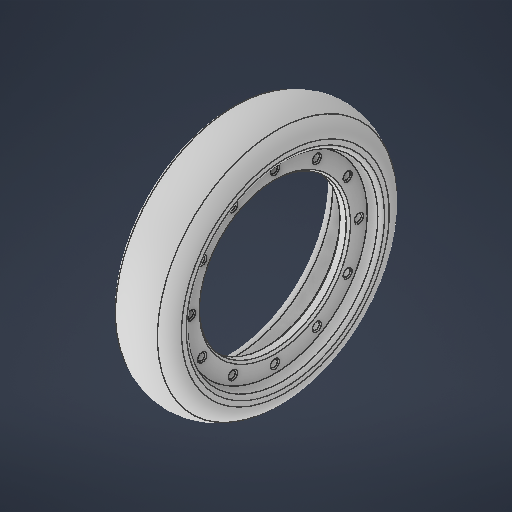
# Autodesk Inventor part: Колесо
Saved by Autodesk Inventor 2025 (Build 290162010, 162A)
## iProperties
Created: 2024-06-21
Part Number: Колесо
Material: Типовые
Document SubType Name: Modeling
Designer: Edward_Higgins
Density: 1 g/cm^3
Appearance: По умолчанию
Author: Edward_Higgins
Autodesk Inventor part; units mm, degrees
ref_plane "YZ Plane" through (0, 0, 0) normal (1, 0, 0) x (0, 1, 0)
ref_plane "XZ Plane" through (0, 0, 0) normal (0, 1, 0) x (-1, 0, 0)
ref_plane "XY Plane" through (0, 0, 0) normal (0, 0, 1) x (1, 0, 0)
sketch "Эскиз1" plane through (0, 0, 0) normal (0, 0, 1) x (1, 0, 0)
  line L0 (0, 0) -> (-61.3454, 0) construction
  line L1 (-14.2142, 60) -> (14.2142, 60) construction
  arc A0 (10, 56.9666) -> (-10, 56.9666) centre (0, 42) ccw
  arc A1 (14, 49.4833) -> (10, 56.9666) centre (5, 49.4833) ccw
  arc A2 (-10, 56.9666) -> (-13.9946, 49.7954) centre (-5, 49.4833) ccw
  line L2 (-3, 0) -> (-3, 9.8)
  line L3 (-3, 9.8) -> (-4.5, 9.8)
  line L4 (-4.5, 9.8) -> (-4.5, 12.1237)
  arc A3 (-3.7958, 13.6471) -> (-1, 18.6167) centre (-9.1319, 19.9203) ccw
  line L5 (4, 0) -> (4, 15)
  line L6 (-3, 4.05) -> (0, 4.05)
  line L7 (0, 4.05) -> (0, 0)
  arc A4 (-3.7958, 13.6471) -> (-4.5, 12.1237) centre (-2.5, 12.1237) ccw
  line L8 (4, 0) -> (-3, 0)
  line L9 (0, 4.05) -> (4, 4.05)
  arc A5 (-13.9946, 49.7954) -> (-9.8383, 46.3489) centre (-10.5856, 49.6771) ccw
  arc A6 (-1.893, 44.4558) -> (-9.8383, 46.3489) centre (-7.8016, 37.2774) ccw
  line L10 (14, 47.2203) -> (14, 49.4833)
  line L11 (9, 35) -> (4, 35)
  line L12 (4, 35) -> (4, 44)
  line L13 (-0.622, 44) -> (4, 44)
  line L14 (4, 15) -> (4, 43.7)
  arc A7 (-0.0249, 35.1197) -> (0, 35.6178) centre (-5, 35.6178) ccw
  arc A8 (-1.893, 44.4558) -> (-0.622, 44) centre (-0.622, 46) ccw
  line L15 (-9.8383, 46.3489) -> (-1.8928, 49.4771)
  arc A9 (0.1678, 45.7397) -> (-1.8928, 49.4771) centre (-1.1045, 47.4749) ccw
  line L16 (0.1678, 45.7397) -> (-0.622, 45.1605)
  line L17 (-0.622, 45.1605) -> (-0.622, 44)
  line L18 (9, 35) -> (9, 44)
  line L19 (9, 44) -> (12.684, 45.3409)
  arc A10 (12.684, 45.3409) -> (14, 47.2203) centre (12, 47.2203) ccw
  point P0 (0, 60)
  point P1 (-4.5, 13.1106)
  point P2 (-1.3791, 44)
  point P3 (0, 0)
  point P4 (14, 45.8199)
  dimension "d1" = 120
  dimension "d4" = 19.6
  dimension "d18" = 8.1
  dimension "d19" = 1.5
  dimension "d20" = 3
  dimension "d21" = 18
  dimension "d22" = 7
  dimension "d24" = 9
  dimension "d26" = 2
  dimension "d27" = 3
  dimension "d46" = 10
  dimension "d47" = 30
  dimension "d83" = 2
  dimension "d106" = 88
  dimension "d118" = 5
  dimension "d119" = 9
  dimension "d120" = 70
  dimension "d121" = 2
  constraints: 40 end point, 25 point on circle, 14 tangent, 11 centre point, 9 point on line, 6 perpendicular, 5 vertical, 4 horizontal, 2 horizontal alignment, 1 equal radius, 1 midpoint, 1 vertical alignment
  measures "d1" diameter of L1 L0
  measures "d4" diameter of L3 L0
  measures "d18" diameter of L6 L0
  measures "d19" distance between parallel lines of L2 L4
  measures "d20" distance between parallel lines of L2 L7
  measures "d21" radius of A0
  measures "d22" distance between parallel lines of L5 L2
  measures "d24" radius of A1
  measures "d26" radius of A4
  measures "d27" distance from line of L0.start L2
  measures "d46" distance of A1.centre A2.centre
  measures "d47" diameter of L5.end L0
  measures "d83" radius of A8
  measures "d106" diameter of L13 L0
  measures "d118" distance between parallel lines of L18 L14
  measures "d119" distance of L11.start L18.end
  measures "d120" angle of L18 L19
  measures "d121" radius of A10
revolve "Вращение1" add sketch "Эскиз1" angle 360 about axis through (0, 0, 0) along (-1, 0, 0) contours A1 L10 A10 L19 L18 L11 L12 L13 L17 L16 A9 L15 A5 A2 A0 | L15 A9 L16 L17 A8 A6
sketch "Эскиз8" plane through (14, 0, 0) normal (1, 0, 0) x (0, 0, -1)
  circle A0 centre (0, -40) radius 3.25
  circle A1 centre (0, -40) radius 1.7
  point P0 (0, 0)
  dimension "d80" = 40
  dimension "d81" = 6.5
  dimension "d82" = 3.4
  constraints: 2 centre point, 1 coincident, 1 vertical alignment
  measures "d80" distance of A0.centre point (0, 0)
  measures "d81" diameter of A0
  measures "d82" diameter of A1
extrude "Выдавливание9" cut sketch "Эскиз8" against normal up to surface (10 mm away) contours A1
chamfer "Фаска6" distance 0.5 angle 45 2 edges at (9, -40, 1.7) (4, -40, 1.7)
pattern_circular "Круговой массив7" count 12 over 360 about axis through (6.5, 0, 0) along (-1, 0, 0) of "Выдавливание9", "Фаска6"
chamfer "Фаска4" distance 1 angle 45 2 edges at (9, -35, 0) (4, -35, 0)
